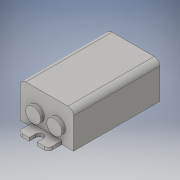
# Autodesk Inventor part: LED Driver
Saved by Autodesk Inventor 2016 (Build 200138000, 138)
## iProperties
Created: 2017-10-25
Part Number: LED Driver
Material: Generic
Document SubType Name: Modeling
Designer: Student
Density: 1 g/cm^3
Appearance: Default
Author: Student
Autodesk Inventor part; units mm, degrees
ref_plane "YZ Plane" through (0, 0, 0) normal (1, 0, 0) x (0, 1, 0)
ref_plane "XZ Plane" through (0, 0, 0) normal (0, 1, 0) x (-1, 0, 0)
ref_plane "XY Plane" through (0, 0, 0) normal (0, 0, 1) x (1, 0, 0)
sketch "Sketch1" plane through (0, 0, 0) normal (0, 1, 0) x (-1, 0, 0)
  line L0 (10.3823, 13.6045) -> (-19.4881, 13.6045)
  line L1 (-19.4881, 13.6045) -> (-19.4881, -34.6555)
  line L2 (-19.4881, -34.6555) -> (10.3823, -34.6555)
  line L3 (10.3823, -34.6555) -> (10.3823, 13.6045)
  point P0 (0, 0)
  dimension "d0" = 48.26
  dimension "d1" = 29.8704
  constraints: 8 end point, 2 parallel, 1 horizontal, 1 perpendicular
  measures "d0" distance of L2.end L0.start
  measures "d1" distance of L1.end L2.end
extrude "Extrusion1" add sketch "Sketch1" along normal blind 20.193
fillet "Fillet1" radius 3.175 2 edges at (19.4881, 20.193, -10.5255) (-10.3823, 20.193, -10.5255)
sketch "Sketch2" plane through (0, 0, 0) normal (0, -1, 0) x (1, 0, 0)
  line L0 (13.0111, -34.6555) -> (13.0111, -42.2755)
  line L1 (19.4881, 13.6045) -> (19.4881, -34.6555) projected
  line L2 (13.0111, -42.2755) -> (6.7881, -42.2755)
  line L3 (6.7881, -42.2755) -> (6.7881, -34.6555)
  line L4 (6.7881, -36.6113) -> (2.3177, -36.6113)
  line L5 (2.3177, -34.6555) -> (2.3177, -42.2755)
  line L6 (2.3177, -42.2755) -> (-3.9053, -42.2755)
  line L7 (-3.9053, -42.2755) -> (-3.9053, -34.6555)
  line L8 (-10.3823, -34.6555) -> (-10.3823, 13.6045) projected
  line L9 (19.4881, -10.5255) -> (-10.3823, -10.5255) construction
  line L10 (13.0111, 13.6045) -> (13.0111, 21.2245)
  line L11 (13.0111, 21.2245) -> (6.7881, 21.2245)
  line L12 (6.7881, 21.2245) -> (6.7881, 13.6045)
  line L13 (6.7881, 15.5603) -> (2.3177, 15.5603)
  line L14 (2.3177, 13.6045) -> (2.3177, 21.2245)
  line L15 (2.3177, 21.2245) -> (-3.9053, 21.2245)
  line L16 (-3.9053, 21.2245) -> (-3.9053, 13.6045)
  line L17 (13.0111, -34.6555) -> (6.7881, -34.6555)
  line L18 (2.3177, -34.6555) -> (-3.9053, -34.6555)
  line L19 (19.4881, -34.6555) -> (-10.3823, -34.6555) projected
  line L20 (6.7881, -34.6555) -> (2.3177, -34.6555)
  line L21 (13.0111, 13.6045) -> (6.7881, 13.6045)
  line L22 (-10.3823, 13.6045) -> (19.4881, 13.6045) projected
  line L23 (6.7881, 13.6045) -> (2.3177, 13.6045)
  line L24 (2.1667, 13.6045) -> (-3.9053, 13.6045)
  line L25 (6.7881, 13.6045) -> (2.3177, 13.6045)
  line L26 (2.3177, 13.6045) -> (2.3177, 15.5603)
  line L27 (2.3177, 15.5603) -> (6.7881, 15.5603)
  line L28 (6.7881, 15.5603) -> (6.7881, 13.6045)
  line L29 (6.7881, -36.6113) -> (2.3177, -36.6113)
  line L30 (2.3177, -36.6113) -> (2.3177, -34.6555)
  line L31 (2.3177, -34.6555) -> (6.7881, -34.6555)
  line L32 (6.7881, -34.6555) -> (6.7881, -36.6113)
  line L33 (-3.9053, 13.6045) -> (2.3177, 13.6045)
  line L34 (2.3177, 13.6045) -> (2.3177, 21.2245)
  line L35 (2.3177, 21.2245) -> (-3.9053, 21.2245)
  line L36 (-3.9053, 21.2245) -> (-3.9053, 13.6045)
  point P0 (0, 0)
  dimension "d5" = 6.477
  dimension "d6" = 7.62
  dimension "d7" = 6.223
  dimension "d9" = 4.4704
  dimension "d10" = 6.223
  dimension "d11" = 7.62
  dimension "d12" = 29.8704
  dimension "d13" = 4.4704
  dimension "d15" = 6.477
  dimension "d16" = 6.477
  dimension "d17" = 6.477
  constraints: 66 end point, 10 symmetric about line, 6 parallel, 5 collinear, 5 horizontal, 5 perpendicular, 4 vertical, 3 point on line, 2 midpoint
  measures "d5" distance between parallel lines of L1 L0
  measures "d6" distance of L0.start L0.end
  measures "d7" distance of L0.end L2.end
  measures "d9" distance of L4.start L4.end
  measures "d10" distance of L5.end L6.end
  measures "d11" distance of L5.start L5.end
  measures "d12" distance between parallel lines of L8 L1
  measures "d13" distance between parallel lines of L5 L3
  measures "d15" distance between parallel lines of L1 L10
  measures "d16" distance between parallel lines of L8 L16
  measures "d17" distance between parallel lines of L7 L8
extrude "Extrusion2" add sketch "Sketch2" against normal blind 1.8542 contours L0 L2 L3 L17 | L3 L4 L5 L19 | L5 L6 L7 L18 | L21 L12 L11 L10 | L22 L14 L13 L12 | L22 L16 L15 L14
fillet "Fillet2" radius 2.2352 4 edges at (6.7881, 0.9271, 15.5603) (2.3177, 0.9271, 15.5603) (6.7881, 0.9271, -36.6113) (2.3177, 0.9271, -36.6113)
fillet "Fillet3" radius 2.2352 4 edges at (-3.9053, 0.9271, -42.2755) (13.0111, 0.9271, -42.2755) (13.0111, 0.9271, 21.2245) (-3.9053, 0.9271, 21.2245)
sketch "Sketch3" plane through (16.3131, 20.193, -34.6555) normal (0, 0, -1) x (-1, 0, 0)
  circle A0 centre (5.5372, -11.9126) radius 4.2418
  circle A1 centre (17.3736, -11.9126) radius 4.2418
  line L0 (20.2184, -20.193) -> (26.6954, -20.193) projected
  line L1 (-3.175, -20.193) -> (3.302, -20.193) projected
  line L2 (-3.175, -20.193) -> (-3.175, -3.175) projected
  line L3 (26.6954, -20.193) -> (26.6954, -3.175) projected
  point P0 (16.3131, -20.193)
  dimension "d22" = 8.4836
  dimension "d23" = 8.4836
  dimension "d24" = 8.2804
  dimension "d25" = 8.2804
  dimension "d26" = 11.8364
  dimension "d27" = 4.4704
  dimension "d28" = 5.08
  constraints: 2 centre point
  measures "d22" diameter of A1
  measures "d23" diameter of A0
  measures "d24" distance from line of L0 A1.centre
  measures "d25" distance from line of L1 A0.centre
  measures "d26" distance of A1.centre A0.centre
  measures "d27" distance edge to line of A0 L2
  measures "d28" distance edge to line of A1 L3
extrude "Extrusion3" add sketch "Sketch3" along normal blind 2.0066 and the other way blind 50.2666
equation "\"d10\" = d7"
equation "\"d11\" = d6"
equation "\"d13\" = d9"
equation "\"d23\" = d22"
equation "\"d25\" = d24"
body "Solid1"
